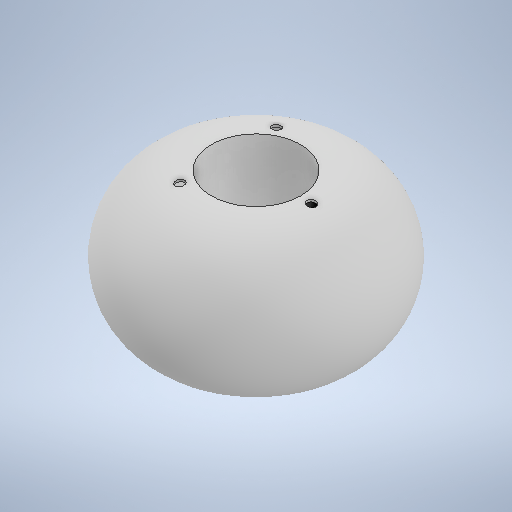
# Autodesk Inventor part: Buoy 6 FatHalfSphere
Saved by Autodesk Inventor 2025 (Build 290162000, 162)
## iProperties
Created: 2024-06-27
Part Number: Buoy 6 FatHalfSphere
Material: Generic
Document SubType Name: Modeling
Designer: track
Density: 1 g/cm^3
Appearance: Default
Author: track
## iProperties of the stored document Buoy 6 FatHalfSphere_3DPrint.ipt
Created: 2024-06-28
Part Number: Buoy 6 FatHalfSphere_3DPrint
Material: Generic
Document SubType Name: Modeling
Designer: track
Density: 1 g/cm^3
Appearance: Default
Author: track
Autodesk Inventor part; units mm, degrees
ref_plane "YZ Plane" through (0, 0, 0) normal (1, 0, 0) x (0, 1, 0)
ref_plane "XZ Plane" through (0, 0, 0) normal (0, 1, 0) x (-1, 0, 0)
ref_plane "XY Plane" through (0, 0, 0) normal (0, 0, 1) x (1, 0, 0)
sketch "Sketch1" plane through (0, 0, 0) normal (0, 0, 1) x (1, 0, 0)
  line L0 (0, 0) -> (0, 101.6) construction
  line L1 (0, 101.6) -> (30.48, 101.6) construction
  line L2 (30.48, 101.6) -> (30.48, 0)
  arc A0 (30.48, 0) -> (30.48, 101.6) centre (30.48, 50.8) ccw
  line L3 (31.98, 1.5228) -> (31.98, 100.0772)
  arc A1 (31.98, 1.5228) -> (31.98, 100.0772) centre (30.48, 50.8) ccw
  dimension "d0" = 30.48
  dimension "d1" = 101.6
  dimension "d2" = 50.8
  dimension "d3" = 1.5
  constraints: 8 end point, 4 point on circle, 2 centre point, 2 perpendicular, 1 tangent, 1 vertical, 1 other
  measures "d0" distance between parallel lines of L2 L0
  measures "d1" distance of L0.start L0.end
  measures "d2" radius of A0
  measures "d3" radial gap between concentric circles of A0 A1
revolve "Revolution1" add sketch "Sketch1" angle 360 about axis through (0, 0, 0) along (0, 1, 0)
sketch "Sketch2" plane through (0, 0, 0) normal (0, 1, 0) x (-1, 0, 0)
  line L0 (0, 0) -> (-38.1, 0) construction
  circle A0 centre (-38.1, 0) radius 3
  dimension "d5" = 6
  dimension "d6" = 38.1
  constraints: 2 end point, 1 centre point, 1 coincident, 1 horizontal
  measures "d5" diameter of A0
  measures "d6" distance of L0.start L0.end
extrude "Extrusion1" cut sketch "Sketch2" along normal blind 101.6
pattern_circular "Circular Pattern1" count 3 over 360 about axis through (0, 50.8, 0) along (0, 1, 0) of "Extrusion1"
body "Solid1"
